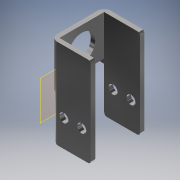
# Autodesk Inventor part: Inline Cylinder Mount Bracket
Saved by Autodesk Inventor 2017 (Build 210142000, 142)
## iProperties
Created: 2016-10-02
Part Number: Inline Cylinder Mount Bracket
Material: Steel, Alloy
Document SubType Name: Modeling
Designer: Aditya
Density: 7.73 g/cm^3
Appearance: Semi-Polished
Author: Aditya
Autodesk Inventor part; units mm, degrees
ref_plane "YZ Plane" through (0, 0, 0) normal (1, 0, 0) x (0, 1, 0)
ref_plane "XZ Plane" through (0, 0, 0) normal (0, 1, 0) x (-1, 0, 0)
ref_plane "XY Plane" through (0, 0, 0) normal (0, 0, 1) x (1, 0, 0)
sketch "Sketch1" plane through (0, 0, 0) normal (1, 0, 0) x (0, 1, 0)
  line L0 (0, 0) -> (0, -25.4)
  line L1 (0, -25.4) -> (25.4, -25.4)
  line L2 (25.4, -25.4) -> (25.4, 0)
  line L3 (25.4, 0) -> (0, 0)
  line L4 (0, 0) -> (0, 2.54)
  line L5 (0, 2.54) -> (25.4, 2.54)
  line L6 (25.4, 2.54) -> (25.4, 0)
  line L7 (0, -25.4) -> (0, -27.94)
  line L8 (0, -27.94) -> (25.4, -27.94)
  line L9 (25.4, -27.94) -> (25.4, -25.4)
  circle A0 centre (13.97, -12.7) radius 7.62
  dimension "d0" = 25.4
  dimension "d1" = 25.4
  dimension "d2" = 2.54
  dimension "d3" = 2.54
  constraints: 20 end point, 6 perpendicular, 2 point on line, 2 vertical, 1 centre point, 1 parallel
  measures "d0" distance of L0.start L0.end
  measures "d1" distance of L0.end L1.end
  measures "d2" distance of L0.start L4.end
  measures "d3" distance of L0.end L7.end
ref_plane "Work Plane2" through (2.54, 0, 0) normal (1, 0, 0) x (0, 0, -1)
sketch "Sketch2" plane through (2.54, 0, 0) normal (1, 0, 0) x (0, 0, -1)
  line L0 (27.94, 25.4) -> (-2.54, 25.4) projected
  line L1 (0, 25.4) -> (0, 0)
  line L2 (-2.54, 25.4) -> (0, 25.4)
  line L3 (-2.54, 25.4) -> (-2.54, 0)
  line L4 (25.4, 0) -> (25.4, 25.4)
  line L5 (27.94, 0) -> (27.94, 25.4) projected
  line L6 (25.4, 25.4) -> (27.94, 25.4)
  line L7 (27.94, 25.4) -> (27.94, 0)
  line L8 (25.4, 0) -> (25.4, -25.4)
  line L9 (25.4, -25.4) -> (27.94, -25.4)
  line L10 (27.94, -25.4) -> (27.94, 0)
  line L11 (-2.54, 0) -> (-2.54, -25.4)
  line L12 (-2.54, -25.4) -> (0, -25.4)
  line L13 (0, -25.4) -> (0, 0)
  dimension "d10" = 2.54
  dimension "d11" = 25.4
  dimension "d12" = 25.4
  constraints: 24 end point, 7 perpendicular, 2 horizontal, 2 point on line, 2 vertical, 1 collinear
  measures "d10" distance of L5.start L4.start
  measures "d11" distance of L4.start L8.end
  measures "d12" distance of L3.end L11.end
extrude "Extrusion2" add sketch "Sketch2" along normal blind 20.32
extrude "Extrusion3" add sketch "Sketch1" along normal blind 2.54
sketch "Sketch3" plane through (2.54, -25.4, 2.54) normal (0, 0, 1) x (1, 0, 0)
  line L0 (0, 0) -> (0, 25.4) projected
  circle A0 centre (5.08, 15.24) radius 2.54
  circle A1 centre (15.24, 15.24) radius 2.54
  point P0 (-2.54, 25.4)
  constraints: 2 centre point
extrude "Extrusion4" cut sketch "Sketch3" against normal blind 40.3225
fillet "Fillet1" radius 1.5875 1 edges at (22.86, -25.4, 1.27)
fillet "Fillet2" radius 1.5875 1 edges at (22.86, -25.4, -26.67)
fillet "Fillet3" radius 1.5875 1 edges at (22.86, 25.4, 1.27)
fillet "Fillet4" radius 1.5875 1 edges at (22.86, 25.4, -26.67)
fillet "Fillet5" radius 1.5875 2 edges at (2.54, -25.4, 1.27) (2.54, -25.4, -26.67)
fillet "Fillet6" radius 3.81 2 edges at (0, 12.7, -27.94) (0, 12.7, 2.54)
sketch "Sketch4" plane through (2.54, 0, -25.4) normal (0, -1, 0) x (1, 0, 0)
  line L0 (0, 25.4) -> (0, 0) projected
  line L1 (0, 25.4) -> (0, 0)
  line L2 (0, 0) -> (-2.54, 0)
  line L3 (-2.54, 0) -> (-2.54, 25.4)
  line L4 (-2.54, 25.4) -> (0, 25.4)
  constraints: 8 end point, 3 perpendicular, 1 collinear
extrude "Extrusion5" cut sketch "Sketch4" against normal blind 2.54
sketch "Sketch5" plane through (22.86, -23.8125, -27.94) normal (0, 0, -1) x (-1, 0, 0)
  line L0 (22.86, 26.3525) -> (22.86, 49.2125) projected
  line L1 (0, 47.625) -> (0, 0) projected
  line L2 (19.05, 49.2125) -> (19.05, -1.5554) projected
  circle A0 centre (9.525, 37.7825) radius 2.3812
  point P0 (22.86, 23.8125)
  dimension "d35" = 4.7625
  constraints: 1 centre point
  measures "d35" diameter of A0
extrude "Extrusion6" cut sketch "Sketch5" against normal blind 38.735
body "Solid1"
